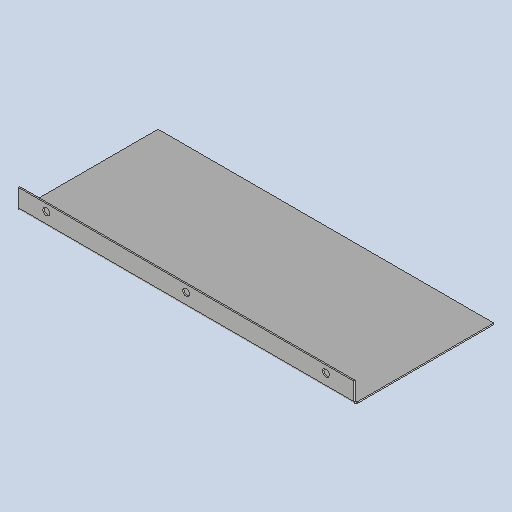
# Autodesk Inventor part: TRM 014 face main
Saved by Autodesk Inventor 2025 (Build 290162010, 162A)
## iProperties
Created: 2024-08-07
Part Number: TRM 014 face main
Material: AISI 304
Document SubType Name: Sheet Metal
Designer: pokla
Density: 8.02768 g/cm^3
Flat Pattern Width: 48 cm
Flat Pattern Length: 22.6202 cm
Flat Pattern Area: 1085.77 cm^2
Sheet Metal Rule: AISI304 2mm Die16
Sheet Metal Width: 480.000 mm
Sheet Metal Length: 226.202 mm
Sheet Metal Area: 108576.956 mm^2
Appearance: Default
Stock Number: ТРМ 014 лицо основное
Mass: 1740.91 g
Surface Area: 2198.78 cm^2
Volume: 216.864 cm^3
Author: pokla
Autodesk Inventor part; units mm, degrees
ref_plane "YZ Plane" through (0, 0, 0) normal (1, 0, 0) x (0, 1, 0)
ref_plane "XZ Plane" through (0, 0, 0) normal (0, 1, 0) x (-1, 0, 0)
ref_plane "XY Plane" through (0, 0, 0) normal (0, 0, 1) x (1, 0, 0)
sketch "Sketch1" plane through (0, 0, 0) normal (0, 0, 1) x (1, 0, 0)
  line L0 (-240, -100) -> (240, -100)
  line L1 (240, -100) -> (240, 100)
  line L2 (240, 100) -> (-240, 100)
  line L3 (-240, 100) -> (-240, -100)
  line L4 (-240, -100) -> (240, 100) construction
  line L5 (240, -100) -> (-240, 100) construction
  point P0 (0, 0)
  dimension "d0" = 480
  dimension "d1" = 200
  measures "d0" distance of L2.end L1.end
  measures "d1" distance of L1.end L0.end
extrude "Plate1" add sketch "Sketch1" along normal blind 2
sketch "Sketch2" plane through (0, 0, 0) normal (0, 0, -1) x (-1, 0, 0)
  line L0 (-220, 80) -> (-20, 80) construction
  line L1 (-20, 80) -> (-20, 60) construction
  line L2 (-20, 60) -> (-220, 60) construction
  line L3 (-220, 60) -> (-220, 80) construction
  line L4 (-240, 100) -> (240, 100) projected
  line L5 (-240, -100) -> (-240, 100) projected
  point P0 (0, 0)
  dimension "d6" = 200
  dimension "d9" = 20
  dimension "d10" = 20
  dimension "d11" = 20
  constraints: 2 other
  measures "d6" distance of L0.start L0.end
  measures "d9" distance of L0.end L1.end
  measures "d10" distance between parallel lines of L4 L0
  measures "d11" distance between parallel lines of L5 L3
mark "Mark1"
sketch "Sketch3" plane through (240, -98, 0) normal (0, -1, 0) x (1, 0, 0)
  line L0 (-480, 0) -> (0, 0)
  line L1 (0, 0) -> (0, 30)
  line L2 (0, 30) -> (-480, 30)
  line L3 (-480, 30) -> (-480, 0)
  constraints: 6 end point, 1 horizontal, 1 perpendicular, 1 vertical
edge flange "Flange1" height 30 angle 90 thickness 2 bend radius 2.75 thickness toward (0, -1, 0) relief round relief width 2 relief depth 1 edges at (0, -100, 2) wall of the first edge with corners at (-240, -98, 0) (240, -98, 0) (240, -98, 30) (-240, -98, 30)
bend "Bend1"
corner "Corner1"
sketch "Sketch4" plane through (-240, -98, 30) normal (0, 1, 0) x (1, 0, 0)
  line L0 (480, 25.25) -> (0, 25.25) projected
  line L1 (0, 25.25) -> (0, 0) projected
  line L2 (0, 0) -> (480, 0) projected
  line L3 (480, 25.25) -> (480, 0) projected
  circle A0 centre (240, 10) radius 5
  point P0 (240, 30)
  point P1 (240, 25.25)
  point P2 (240, 0)
  dimension "d22" = 10
  dimension "d23" = 10
  constraints: 2 midpoint, 1 centre point, 1 vertical alignment
  measures "d22" diameter of A0
  measures "d23" distance of point (240, 0) A0.centre
extrude "Cut1" cut sketch "Sketch4" against normal blind 2 contours A0
pattern_linear "Rectangular Pattern1" count 3 spacing 200 along (1, 0, 0) of "Cut1" first direction both ways yes
equation "\"d24\" = Thickness"
equation "\"d2\" = Thickness"
equation "\"d12\" = BendReliefWidth"
equation "\"d13\" = BendReliefDepth"
equation "\"d14\" = MinimumRemnant"
equation "\"d15\" = TransitionRadius"
equation "\"d18\" = BendRadius"
equation "\"d19\" = CornerReliefSize"
equation "\"d20\" = GapSize"
equation "\"d21\" = JacobiRadiusSize"
equation "\"BendReliefWidth\" = Thickness"
equation "\"BendReliefDepth\" = 0.5 * Thickness"
equation "\"CornerReliefSize\" = 4 * Thickness"
equation "\"MinimumRemnant\" = 2 * Thickness"
equation "\"TransitionRadius\" = BendRadius"
equation "\"JacobiRadiusSize\" = BendRadius"
equation "\"GapSize\" = Thickness"
equation "\"Thickness\" = 2"
equation "\"BendRadius\" = 2.75"
body "Solid1"
